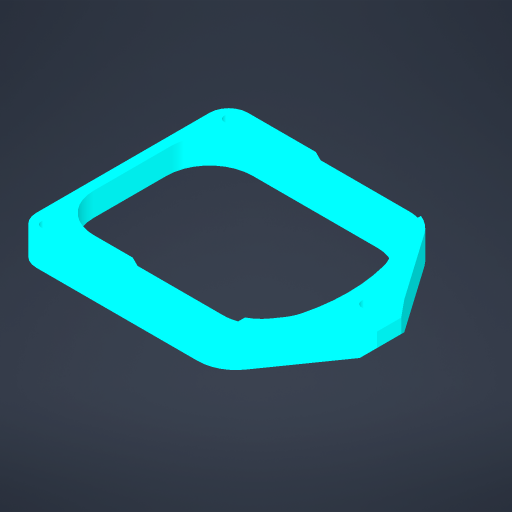
# Autodesk Inventor part: X Stage Part V5
Saved by Autodesk Inventor 2023.4 (Build 274418000, 418)
## iProperties
Created: 2024-05-20
Part Number: X Stage Part V5
Material: Generic
Document SubType Name: Modeling
Designer: xSibe
Density: 1 g/cm^3
Appearance: Plastic Cyan
Author: xSibe
Autodesk Inventor part; units mm, degrees
ref_plane "YZ Plane" through (0, 0, 0) normal (1, 0, 0) x (0, 1, 0)
ref_plane "XZ Plane" through (0, 0, 0) normal (0, 1, 0) x (-1, 0, 0)
ref_plane "XY Plane" through (0, 0, 0) normal (0, 0, 1) x (1, 0, 0)
sketch "Sketch1" plane through (0, 0, 0) normal (0, 1, 0) x (-1, 0, 0)
  circle A0 centre (-61.4078, 0) radius 1.5625 projected
  line L0 (-67.0776, 3.125) -> (-65.2026, 3.125) projected
  arc A1 (-60.6131, 4.375) -> (-67.0776, 3.125) centre (-60.6131, -12.9657) ccw projected
  arc A2 (-57.9614, 3.2767) -> (-60.6131, 4.375) centre (-60.6131, 0.625) ccw projected
  line L1 (-57.9614, 3.2767) -> (-57.3364, 2.6516) projected
  arc A3 (-57.3364, -2.6516) -> (-57.3364, 2.6516) centre (-59.9881, 0) ccw projected
  line L2 (-57.3364, -2.6516) -> (-57.9614, -3.2767) projected
  arc A4 (-60.6131, -4.375) -> (-57.9614, -3.2767) centre (-60.6131, -0.625) ccw projected
  arc A5 (-67.0776, -3.125) -> (-60.6131, -4.375) centre (-60.6131, 12.9657) ccw projected
  line L3 (-65.2026, -3.125) -> (-67.0776, -3.125) projected
  line L4 (-65.2026, 3.125) -> (-65.2026, -3.125) projected
  line L5 (-65.2026, -3.125) -> (-67.0776, -3.125) projected
  line L6 (-67.0776, -3.125) -> (-67.0776, 3.125) projected
  line L7 (-67.0776, 3.125) -> (-65.2026, 3.125) projected
  line L8 (-65.2026, 3.125) -> (-65.2026, -3.125) projected
  line L9 (-67.0776, -3.125) -> (-58.4739, -15.4123)
  line L10 (-58.4739, -15.4123) -> (-54.3781, -12.5444)
  line L11 (-54.3781, -12.5444) -> (-62.9818, -0.2571)
  line L12 (-62.9818, -0.2571) -> (-67.0776, -3.125)
  line L13 (-67.0776, -3.125) -> (-52.0776, -3.125) construction
  line L14 (-67.0776, 0) -> (-65.2026, 0)
  line L15 (-67.0776, 3.125) -> (-58.4739, 15.4123)
  line L16 (-58.4739, 15.4123) -> (-54.3781, 12.5444)
  line L17 (-54.3781, 12.5444) -> (-62.9818, 0.2571)
  line L18 (-62.9818, 0.2571) -> (-67.0776, 3.125)
  arc A6 (-54.3781, 12.5444) -> (-54.3781, -12.5444) centre (-13.0052, 0) ccw
  point P0 (0, 0)
  dimension "d0" = 15
  dimension "d1" = 55
  dimension "d2" = 5
  constraints: 20 end point, 3 symmetric about line, 2 midpoint, 2 parallel, 2 point on circle, 1 centre point, 1 equal length, 1 horizontal, 1 perpendicular, 1 tangent
  measures "d0" distance of L3.end L9.end
  measures "d1" angle of L9 L13
  measures "d2" distance of L10.end L9.end
ref_plane "Work Plane1" through (56.2381, 16.5156, -3.125) normal (0, 1, 0) x (0, 0, 1)
ref_plane "Work Plane2" through (54.9881, 24.0156, -4.375) normal (0, -1, 0) x (1, 0, 0)
extrude "Extrusion1" add sketch "Sketch1" along normal up to surface (7.5 mm away) from surface at 16.5156 contours A0 L17 A2 L1 A3 L2 A4 L11 | A0 L17 L18 L4 L0 A1 A2 | L11 A4 A5 L3 L4 L12 A0 | A0 L11 L12 L4 L18 L17 | L17 A6 A3 L1 A2 | A2 A1 L15 L16 L17 | L11 L10 L9 A5 A4 | A4 L2 A3 A6 L11 | L18 L0 L4 | L4 L14 L6 L18 | L12 L6 L14 L4 | L4 L3 L12
chamfer "Chamfer1" distance 1.875 angle 45 2 edges at (67.0776, 24.0156, 0) (67.0776, 16.5156, 0)
sketch "Sketch2" plane through (0, 0, 0) normal (0, 0, 1) x (1, 0, 0)
  line L0 (67.0776, 18.3906) -> (65.2026, 16.5156) projected
  line L1 (67.0776, 18.3906) -> (67.0776, 22.1406) projected
  line L2 (65.2026, 24.0156) -> (67.0776, 22.1406) projected
  line L3 (58.4739, 24.0156) -> (65.2026, 24.0156) projected
  line L4 (58.4739, 16.5156) -> (58.4739, 24.0156) projected
  line L5 (65.2026, 16.5156) -> (58.4739, 16.5156) projected
  line L6 (54.3781, 24.0156) -> (58.4739, 24.0156) projected
  line L7 (54.3781, 16.5156) -> (54.3781, 24.0156) projected
  line L8 (58.4739, 16.5156) -> (54.3781, 16.5156) projected
  line L9 (58.4739, 16.5156) -> (58.4739, 24.0156) projected
  line L10 (65.187, 23.9781) -> (67.0401, 22.1251)
  line L11 (67.0401, 22.1251) -> (67.0401, 18.4062)
  line L12 (67.0401, 18.4062) -> (65.187, 16.5531)
  line L13 (65.187, 16.5531) -> (58.5114, 16.5531)
  line L14 (58.5114, 16.5531) -> (58.5114, 23.9781)
  line L15 (58.5114, 23.9781) -> (65.187, 23.9781)
  line L16 (58.4364, 23.9781) -> (54.4156, 23.9781)
  line L17 (54.4156, 23.9781) -> (54.4156, 16.5531)
  line L18 (54.4156, 16.5531) -> (58.4364, 16.5531)
  line L19 (58.4364, 16.5531) -> (58.4364, 23.9781)
  line L20 (54.3781, 23.9781) -> (65.187, 23.9781)
  line L21 (65.187, 16.5531) -> (54.3781, 16.5531)
  point P0 (0, 0)
  dimension "d8" = 0.0375
  dimension "d9" = 0.0375
  constraints: 24 end point, 2 point on line, 1 collinear, 1 perpendicular, 8 other
  measures "d8" distance between parallel lines of L3 L15
  measures "d9" distance between parallel lines of L6 L16
extrude "Extrusion2" cut sketch "Sketch2" along normal mid plane 50 contours L0 L5 L4 L21 L13 L12 L11 L10 L15 L20 L3 L2 L1 | L8 L7 L21 L18 L4 | L4 L20 L16 L7 L6
sketch "Sketch3" plane through (13.0052, 23.9781, 0) normal (0, 1, 0) x (1, 0, 0)
  line L0 (45.4687, 15.4123) -> (52.1818, 5.825) projected
  line L1 (41.373, 12.5444) -> (45.4687, 15.4123) projected
  arc A0 (41.373, -12.5444) -> (41.373, 12.5444) centre (0, 0) ccw projected
  line L2 (45.4687, -15.4123) -> (41.373, -12.5444) projected
  line L3 (52.1818, -5.825) -> (45.4687, -15.4123) projected
  line L4 (52.1818, 5.825) -> (52.1818, -5.825) projected
  circle A1 centre (48.4026, 0) radius 1.5625 projected
  line L5 (45.4687, -15.4123) -> (41.373, -12.5444)
  line L6 (41.373, -12.5444) -> (32.7693, -24.8317)
  line L7 (32.7693, -24.8317) -> (36.8651, -27.6996)
  line L8 (36.8651, -27.6996) -> (45.4687, -15.4123)
  line L9 (36.8651, -27.6996) -> (36.8651, -20.1996)
  line L10 (36.8651, -20.1996) -> (-15.6349, -20.1996)
  line L11 (-15.6349, -20.1996) -> (-15.6349, -27.6996)
  line L12 (-15.6349, -27.6996) -> (36.8651, -27.6996)
  line L13 (36.8651, -27.6996) -> (44.3651, -27.6996) construction
  line L14 (52.1818, 0) -> (48.4026, 0)
  line L15 (45.4687, 15.4123) -> (41.373, 12.5444)
  line L16 (41.373, 12.5444) -> (32.7693, 24.8317)
  line L17 (32.7693, 24.8317) -> (36.8651, 27.6996)
  line L18 (36.8651, 27.6996) -> (45.4687, 15.4123)
  line L19 (36.8651, 27.6996) -> (36.8651, 20.1996)
  line L20 (36.8651, 20.1996) -> (-15.6349, 20.1996)
  line L21 (-15.6349, 20.1996) -> (-15.6349, 27.6996)
  line L22 (-15.6349, 27.6996) -> (36.8651, 27.6996)
  line L23 (-15.6349, -27.6996) -> (-15.6349, 27.6996)
  line L24 (-15.6349, 27.6996) -> (-13.1349, 27.6996)
  line L25 (-13.1349, 27.6996) -> (-13.1349, -27.6996)
  line L26 (-13.1349, -27.6996) -> (-15.6349, -27.6996)
  point P0 (-13.0052, 0)
  point P1 (36.0128, -20.1996)
  point P2 (-13.1349, -20.1996)
  point P3 (-13.1349, 20.1996)
  point P4 (36.0128, 20.1996)
  point P5 (-15.6349, 20.1996)
  dimension "d12" = 15
  dimension "d13" = 7.5
  dimension "d14" = 90
  dimension "d15" = 52.5
  dimension "d16" = 2.5
  constraints: 44 end point, 6 parallel, 5 symmetric about line, 4 perpendicular, 2 collinear, 2 horizontal, 1 midpoint, 1 vertical
  measures "d12" distance of L6.end L2.end
  measures "d13" distance of L7.end L9.end
  measures "d14" angle of L13 L9
  measures "d15" distance of L10.end L9.end
  measures "d16" distance of L22.start L24.end
extrude "Extrusion3" add sketch "Sketch3" against normal up to surface (7.425 mm away) contours L1 L16 L20 L19 L18 | L19 L20 L16 L17 | L17 L16 L20 L25 L22 | L2 L8 L9 L10 L6 | L25 L20 L21 L22 | L10 L9 L7 L6 | L6 L7 L12 L25 L10 | L25 L10 L23 L20 | L25 L12 L11 L10
fillet "Fillet1" radius 10 8 edges at (49.0179, 20.2656, 20.1996) (54.3781, 20.2656, 12.5444) (54.3781, 20.2656, -12.5444) (49.0179, 20.2656, -20.1996) (49.8703, 20.2656, -27.6996) (49.8703, 20.2656, 27.6996) (-0.1297, 20.2656, 20.1996) (-0.1297, 20.2656, -20.1996)
fillet "Fillet2" radius 5 2 edges at (-2.6297, 20.2656, -27.6996) (-2.6297, 20.2656, 27.6996)
sketch "Sketch4" plane through (0, 0, 0) normal (0, 0, 1) x (1, 0, 0)
  line L0 (2.3703, 16.5531) -> (44.6646, 16.5531) projected
  line L1 (44.6646, 23.9781) -> (2.3703, 23.9781) projected
  line L2 (10.15, 2.5) -> (37.65, 2.5) projected
  line L3 (37.65, 0) -> (10.15, 0) projected
  line L4 (23.9, 0) -> (23.9, 2.5)
  line L5 (23.9, 2.5) -> (23.9, 23.9781)
  line L6 (2.3703, 23.9781) -> (2.3703, 16.5531) projected
  line L7 (44.6646, 16.5531) -> (44.6646, 23.9781) projected
  line L8 (44.6646, 23.9781) -> (48.4073, 23.9781)
  line L9 (48.4073, 23.9781) -> (20.1573, 23.9781)
  line L10 (20.1573, 23.9781) -> (20.1573, 22.7281)
  line L11 (20.1573, 22.7281) -> (48.4073, 22.7281)
  line L12 (48.4073, 22.7281) -> (48.4073, 23.9781)
  point P0 (0, 0)
  dimension "d21" = 3.7427
  dimension "d22" = 28.25
  dimension "d23" = 1.25
  constraints: 14 end point, 2 horizontal, 2 midpoint, 2 parallel, 2 point on line, 1 perpendicular
  measures "d21" distance of L1.start L8.end
  measures "d22" distance of L11.end L10.end
  measures "d23" distance of L10.end L9.end
extrude "Extrusion4" cut sketch "Sketch4" along normal up to surface (55.3991 mm away) from surface at -27.6996 contours L11 L10 L1 L5 | L5 L1 L7 L11 | L7 L8 L12 L11
chamfer "Chamfer2" distance 1.25 angle 45 4 edges at (48.4073, 22.7281, -23.027) (48.4073, 22.7281, 23.027) (20.1573, 22.7281, 23.9496) (20.1573, 22.7281, -23.9496)
sketch "Sketch5" plane through (-0.1297, 23.9781, 10.1996) normal (0, 1, 0) x (1, 0, 0)
  line L0 (20.287, -17.5) -> (20.287, -10) projected
  line L1 (20.287, -10) -> (10, -10) projected
  arc A0 (0, 0) -> (10, -10) centre (10, 0) ccw projected
  line L2 (0, 0) -> (0, 20.3991) projected
  arc A1 (10, 30.3991) -> (0, 20.3991) centre (10, 20.3991) ccw projected
  line L3 (10, 30.3991) -> (20.287, 30.3991) projected
  line L4 (20.287, 30.3991) -> (20.287, 37.8991) projected
  line L5 (20.287, 37.8991) -> (2.5, 37.8991) projected
  arc A2 (2.5, 37.8991) -> (-2.5, 32.8991) centre (2.5, 32.8991) ccw projected
  line L6 (-2.5, 32.8991) -> (-2.5, -12.5) projected
  arc A3 (-2.5, -12.5) -> (2.5, -17.5) centre (2.5, -12.5) ccw projected
  line L7 (2.5, -17.5) -> (20.287, -17.5) projected
  line L8 (20.287, -13.75) -> (-2.5, -13.75)
  line L9 (-2.5, 32.8991) -> (-2.5, -12.5) projected
  line L10 (-2.5, -13.75) -> (1.5, -13.75)
  circle A4 centre (1.5, -13.75) radius 1.4375
  line L11 (0, 10.1996) -> (-2.5, 10.1996)
  circle A5 centre (1.5, 34.1491) radius 1.4375
  point P0 (0.1297, 10.1996)
  dimension "d29" = 4
  dimension "d30" = 2.875
  constraints: 6 end point, 3 midpoint, 2 centre point, 2 point on line, 1 coincident, 1 horizontal, 1 symmetric about line, 1 other
  measures "d29" distance of L8.end L10.end
  measures "d30" diameter of A4
extrude "Extrusion5" cut sketch "Sketch5" against normal up to surface (7.425 mm away) contours A4 L8 | L8 A4 | A5
chamfer "Chamfer3" distance 1.25 angle 45 12 edges at (26.8413, 16.5531, -20.1996) (2.7992, 16.5531, -17.2706) (-0.1297, 16.5531, 0) (2.7992, 16.5531, 17.2706) (26.8413, 16.5531, 20.1996) (48.4298, 16.5531, 19.0697) (52.7024, 16.5531, 14.9376) (54.2985, 16.5531, 12.3742) (56.2381, 16.5531, 0) (54.2985, 16.5531, -12.3742) (52.7024, 16.5531, -14.9376) (48.4298, 16.5531, -19.0697)
body "Solid1"
